Autodesk Inventor part; units mm, degrees
(part 4 of 8)
  line L1567 (12.2801, 87.4726) -> (12.299, 87.794) construction
  line L1568 (12.299, 87.794) -> (12.3274, 88.6686) construction
  line L1569 (12.3274, 88.6686) -> (12.3369, 89.0704) construction
  spline S407 degree 2 poles (9.1271, 85.2036) (9.6944, 85.2036) (10.3184, 86.0403) (10.3184, 86.8817) knots 0 0 0 1 2 2 2
  line L1570 (9.1271, 85.2036) -> (9.6944, 85.2036) construction
  line L1571 (9.6944, 85.2036) -> (10.3184, 86.0403) construction
  line L1572 (10.3184, 86.0403) -> (10.3184, 86.8817) construction
  spline S408 degree 2 poles (10.3184, 86.8817) (10.3184, 87.7326) (9.6991, 88.5599) (9.1271, 88.5599) knots 0 0 0 1 2 2 2
  line L1573 (10.3184, 86.8817) -> (10.3184, 87.7326) construction
  line L1574 (10.3184, 87.7326) -> (9.6991, 88.5599) construction
  line L1575 (9.6991, 88.5599) -> (9.1271, 88.5599) construction
  spline S409 degree 2 poles (9.1271, 88.5599) (8.5551, 88.5599) (7.9311, 87.7326) (7.9311, 86.8817) knots 0 0 0 1 2 2 2
  line L1576 (9.1271, 88.5599) -> (8.5551, 88.5599) construction
  line L1577 (8.5551, 88.5599) -> (7.9311, 87.7326) construction
  line L1578 (7.9311, 87.7326) -> (7.9311, 86.8817) construction
  spline S410 degree 2 poles (7.9311, 86.8817) (7.9311, 86.0544) (8.5551, 85.2036) (9.1271, 85.2036) knots 0 0 0 1 2 2 2
  line L1579 (7.9311, 86.8817) -> (7.9311, 86.0544) construction
  line L1580 (7.9311, 86.0544) -> (8.5551, 85.2036) construction
  line L1581 (8.5551, 85.2036) -> (9.1271, 85.2036) construction
  spline S411 degree 2 poles (9.1271, 84.5701) (8.2148, 84.5701) (7.1701, 85.8134) (7.1701, 86.8817) knots 0 0 0 1 2 2 2
  line L1582 (9.1271, 84.5701) -> (8.2148, 84.5701) construction
  line L1583 (8.2148, 84.5701) -> (7.1701, 85.8134) construction
  line L1584 (7.1701, 85.8134) -> (7.1701, 86.8817) construction
  spline S412 degree 2 poles (7.1701, 86.8817) (7.1701, 87.9784) (8.2478, 89.1933) (9.1271, 89.1933) knots 0 0 0 1 2 2 2
  line L1585 (7.1701, 86.8817) -> (7.1701, 87.9784) construction
  line L1586 (7.1701, 87.9784) -> (8.2478, 89.1933) construction
  line L1587 (8.2478, 89.1933) -> (9.1271, 89.1933) construction
  spline S413 degree 2 poles (9.1271, 89.1933) (10.0158, 89.1933) (11.0794, 87.9831) (11.0794, 86.8817) knots 0 0 0 1 2 2 2
  line L1588 (9.1271, 89.1933) -> (10.0158, 89.1933) construction
  line L1589 (10.0158, 89.1933) -> (11.0794, 87.9831) construction
  line L1590 (11.0794, 87.9831) -> (11.0794, 86.8817) construction
  spline S414 degree 2 poles (11.0794, 86.8817) (11.0794, 85.7755) (10.0158, 84.5701) (9.1271, 84.5701) knots 0 0 0 1 2 2 2
  line L1591 (11.0794, 86.8817) -> (11.0794, 85.7755) construction
  line L1592 (11.0794, 85.7755) -> (10.0158, 84.5701) construction
  line L1593 (10.0158, 84.5701) -> (9.1271, 84.5701) construction
  spline S415 degree 2 poles (4.7497, 85.2697) (5.3217, 85.2697) (5.9552, 86.1112) (5.9552, 86.9148) knots 0 0 0 1 2 2 2
  line L1594 (4.7497, 85.2697) -> (5.3217, 85.2697) construction
  line L1595 (5.3217, 85.2697) -> (5.9552, 86.1112) construction
  line L1596 (5.9552, 86.1112) -> (5.9552, 86.9148) construction
  spline S416 degree 2 poles (5.9552, 86.9148) (5.9552, 87.6664) (5.4777, 88.4937) (4.9436, 88.4937) knots 0 0 0 1 2 2 2
  line L1597 (5.9552, 86.9148) -> (5.9552, 87.6664) construction
  line L1598 (5.9552, 87.6664) -> (5.4777, 88.4937) construction
  line L1599 (5.4777, 88.4937) -> (4.9436, 88.4937) construction
  spline S417 degree 2 poles (4.9436, 88.4937) (4.6316, 88.4937) (4.0454, 88.2148) (3.7854, 87.9973) knots 0 0 0 1 2 2 2
  line L1600 (4.9436, 88.4937) -> (4.6316, 88.4937) construction
  line L1601 (4.6316, 88.4937) -> (4.0454, 88.2148) construction
  line L1602 (4.0454, 88.2148) -> (3.7854, 87.9973) construction
  line L1603 (3.7854, 87.9973) -> (3.7854, 85.5108)
  spline S418 degree 2 poles (3.7854, 85.5108) (4.0738, 85.3737) (4.485, 85.2697) (4.7497, 85.2697) knots 0 0 0 1 2 2 2
  line L1604 (3.7854, 85.5108) -> (4.0738, 85.3737) construction
  line L1605 (4.0738, 85.3737) -> (4.485, 85.2697) construction
  line L1606 (4.485, 85.2697) -> (4.7497, 85.2697) construction
  spline S419 degree 2 poles (4.8726, 84.6079) (4.5465, 84.6079) (4.0454, 84.7592) (3.7854, 84.9152) knots 0 0 0 1 2 2 2
  line L1607 (4.8726, 84.6079) -> (4.5465, 84.6079) construction
  line L1608 (4.5465, 84.6079) -> (4.0454, 84.7592) construction
  line L1609 (4.0454, 84.7592) -> (3.7854, 84.9152) construction
  spline S420 degree 2 poles (3.7854, 88.6119) (4.0596, 88.8624) (4.7308, 89.1933) (5.1232, 89.1933) knots 0 0 0 1 2 2 2
  line L1610 (3.7854, 88.6119) -> (4.0596, 88.8624) construction
  line L1611 (4.0596, 88.8624) -> (4.7308, 89.1933) construction
  line L1612 (4.7308, 89.1933) -> (5.1232, 89.1933) construction
  spline S421 degree 2 poles (5.1232, 89.1933) (5.8748, 89.1933) (6.7162, 88.002) (6.7162, 86.9999) knots 0 0 0 1 2 2 2
  line L1613 (5.1232, 89.1933) -> (5.8748, 89.1933) construction
  line L1614 (5.8748, 89.1933) -> (6.7162, 88.002) construction
  line L1615 (6.7162, 88.002) -> (6.7162, 86.9999) construction
  spline S422 degree 2 poles (6.7162, 86.9999) (6.7162, 85.9032) (5.6715, 84.6079) (4.8726, 84.6079) knots 0 0 0 1 2 2 2
  line L1616 (6.7162, 86.9999) -> (6.7162, 85.9032) construction
  line L1617 (6.7162, 85.9032) -> (5.6715, 84.6079) construction
  line L1618 (5.6715, 84.6079) -> (4.8726, 84.6079) construction
  spline S423 degree 2 poles (-7.9191, 85.2036) (-7.3518, 85.2036) (-6.7278, 86.0403) (-6.7278, 86.8817) knots 0 0 0 1 2 2 2
  line L1619 (-7.9191, 85.2036) -> (-7.3518, 85.2036) construction
  line L1620 (-7.3518, 85.2036) -> (-6.7278, 86.0403) construction
  line L1621 (-6.7278, 86.0403) -> (-6.7278, 86.8817) construction
  spline S424 degree 2 poles (-6.7278, 86.8817) (-6.7278, 87.7326) (-7.3471, 88.5599) (-7.9191, 88.5599) knots 0 0 0 1 2 2 2
  line L1622 (-6.7278, 86.8817) -> (-6.7278, 87.7326) construction
  line L1623 (-6.7278, 87.7326) -> (-7.3471, 88.5599) construction
  line L1624 (-7.3471, 88.5599) -> (-7.9191, 88.5599) construction
  spline S425 degree 2 poles (-7.9191, 88.5599) (-8.4911, 88.5599) (-9.1151, 87.7326) (-9.1151, 86.8817) knots 0 0 0 1 2 2 2
  line L1625 (-7.9191, 88.5599) -> (-8.4911, 88.5599) construction
  line L1626 (-8.4911, 88.5599) -> (-9.1151, 87.7326) construction
  line L1627 (-9.1151, 87.7326) -> (-9.1151, 86.8817) construction
  spline S426 degree 2 poles (-9.1151, 86.8817) (-9.1151, 86.0544) (-8.4911, 85.2036) (-7.9191, 85.2036) knots 0 0 0 1 2 2 2
  line L1628 (-9.1151, 86.8817) -> (-9.1151, 86.0544) construction
  line L1629 (-9.1151, 86.0544) -> (-8.4911, 85.2036) construction
  line L1630 (-8.4911, 85.2036) -> (-7.9191, 85.2036) construction
  spline S427 degree 2 poles (-7.9191, 84.5701) (-8.8314, 84.5701) (-9.8761, 85.8134) (-9.8761, 86.8817) knots 0 0 0 1 2 2 2
  line L1631 (-7.9191, 84.5701) -> (-8.8314, 84.5701) construction
  line L1632 (-8.8314, 84.5701) -> (-9.8761, 85.8134) construction
  line L1633 (-9.8761, 85.8134) -> (-9.8761, 86.8817) construction
  spline S428 degree 2 poles (-9.8761, 86.8817) (-9.8761, 87.9784) (-8.7983, 89.1933) (-7.9191, 89.1933) knots 0 0 0 1 2 2 2
  line L1634 (-9.8761, 86.8817) -> (-9.8761, 87.9784) construction
  line L1635 (-9.8761, 87.9784) -> (-8.7983, 89.1933) construction
  line L1636 (-8.7983, 89.1933) -> (-7.9191, 89.1933) construction
  spline S429 degree 2 poles (-7.9191, 89.1933) (-7.0304, 89.1933) (-5.9668, 87.9831) (-5.9668, 86.8817) knots 0 0 0 1 2 2 2
  line L1637 (-7.9191, 89.1933) -> (-7.0304, 89.1933) construction
  line L1638 (-7.0304, 89.1933) -> (-5.9668, 87.9831) construction
  line L1639 (-5.9668, 87.9831) -> (-5.9668, 86.8817) construction
  spline S430 degree 2 poles (-5.9668, 86.8817) (-5.9668, 85.7755) (-7.0304, 84.5701) (-7.9191, 84.5701) knots 0 0 0 1 2 2 2
  line L1640 (-5.9668, 86.8817) -> (-5.9668, 85.7755) construction
  line L1641 (-5.9668, 85.7755) -> (-7.0304, 84.5701) construction
  line L1642 (-7.0304, 84.5701) -> (-7.9191, 84.5701) construction
  spline S431 degree 2 poles (-1.6305, 79.8157) (-1.4362, 79.8157) (-1.3218, 79.944) knots 0 0 0 1 1 1
  line L1643 (-1.6305, 79.8157) -> (-1.4362, 79.8157) construction
  line L1644 (-1.4362, 79.8157) -> (-1.3218, 79.944) construction
  spline S432 degree 2 poles (-1.3218, 79.944) (-1.2177, 80.062) (-1.2177, 80.232) knots 0 0 0 1 1 1
  line L1645 (-1.3218, 79.944) -> (-1.2177, 80.062) construction
  line L1646 (-1.2177, 80.062) -> (-1.2177, 80.232) construction
  spline S433 degree 2 poles (-1.2177, 80.232) (-1.2177, 80.402) (-1.3218, 80.5165) knots 0 0 0 1 1 1
  line L1647 (-1.2177, 80.232) -> (-1.2177, 80.402) construction
  line L1648 (-1.2177, 80.402) -> (-1.3218, 80.5165) construction
  spline S434 degree 2 poles (-1.3218, 80.5165) (-1.4362, 80.6448) (-1.6305, 80.6448) knots 0 0 0 1 1 1
  line L1649 (-1.3218, 80.5165) -> (-1.4362, 80.6448) construction
  line L1650 (-1.4362, 80.6448) -> (-1.6305, 80.6448) construction
  spline S435 degree 2 poles (-1.6305, 81.0612) (-1.2385, 81.0612) (-1.0095, 80.801) knots 0 0 0 1 1 1
  line L1651 (-1.6305, 81.0612) -> (-1.2385, 81.0612) construction
  line L1652 (-1.2385, 81.0612) -> (-1.0095, 80.801) construction
  spline S436 degree 2 poles (-1.0095, 80.801) (-0.8014, 80.5685) (-0.8014, 80.232) knots 0 0 0 1 1 1
  line L1653 (-1.0095, 80.801) -> (-0.8014, 80.5685) construction
  line L1654 (-0.8014, 80.5685) -> (-0.8014, 80.232) construction
  spline S437 degree 2 poles (-0.8014, 80.232) (-0.8014, 79.8955) (-1.0095, 79.6561) knots 0 0 0 1 1 1
  line L1655 (-0.8014, 80.232) -> (-0.8014, 79.8955) construction
  line L1656 (-0.8014, 79.8955) -> (-1.0095, 79.6561) construction
  spline S438 degree 2 poles (-1.0095, 79.6561) (-1.2385, 79.3994) (-1.6305, 79.3994) knots 0 0 0 1 1 1
  line L1657 (-1.0095, 79.6561) -> (-1.2385, 79.3994) construction
  line L1658 (-1.2385, 79.3994) -> (-1.6305, 79.3994) construction
  line L1659 (-1.6305, 79.3994) -> (-2.255, 79.3994)
  spline S439 degree 2 poles (-2.255, 79.3994) (-2.4632, 79.3994) (-2.4632, 79.6075) knots 0 0 0 1 1 1
  line L1660 (-2.255, 79.3994) -> (-2.4632, 79.3994) construction
  line L1661 (-2.4632, 79.3994) -> (-2.4632, 79.6075) construction
  line L1662 (-2.4632, 79.6075) -> (-2.4632, 82.0985)
  spline S440 degree 2 poles (-2.4632, 82.0985) (-2.4632, 82.3067) (-2.255, 82.3067) knots 0 0 0 1 1 1
  line L1663 (-2.4632, 82.0985) -> (-2.4632, 82.3067) construction
  line L1664 (-2.4632, 82.3067) -> (-2.255, 82.3067) construction
  spline S441 degree 2 poles (-2.255, 82.3067) (-2.0468, 82.3067) (-2.0468, 82.0985) knots 0 0 0 1 1 1
  line L1665 (-2.255, 82.3067) -> (-2.0468, 82.3067) construction
  line L1666 (-2.0468, 82.3067) -> (-2.0468, 82.0985) construction
  spline S442 degree 2 poles (-12.0177, 79.6075) (-12.0177, 79.3994) (-12.2259, 79.3994) knots 0 0 0 1 1 1
  line L1667 (-12.0177, 79.6075) -> (-12.0177, 79.3994) construction
  line L1668 (-12.0177, 79.3994) -> (-12.2259, 79.3994) construction
  spline S443 degree 2 poles (-12.2259, 79.3994) (-12.434, 79.3994) (-12.434, 79.6075) knots 0 0 0 1 1 1
  line L1669 (-12.2259, 79.3994) -> (-12.434, 79.3994) construction
  line L1670 (-12.434, 79.3994) -> (-12.434, 79.6075) construction
  line L1671 (-12.434, 79.6075) -> (-12.434, 82.0985)
  spline S444 degree 2 poles (-12.434, 82.0985) (-12.434, 82.3067) (-12.2259, 82.3067) knots 0 0 0 1 1 1
  line L1672 (-12.434, 82.0985) -> (-12.434, 82.3067) construction
  line L1673 (-12.434, 82.3067) -> (-12.2259, 82.3067) construction
  line L1674 (-12.2259, 82.3067) -> (-10.3559, 82.3067)
  spline S445 degree 2 poles (-10.3559, 82.3067) (-10.0124, 82.3067) (-9.5267, 81.8209) (-9.5267, 81.4775) knots 0 0 0 1 2 2 2
  line L1675 (-10.3559, 82.3067) -> (-10.0124, 82.3067) construction
  line L1676 (-10.0124, 82.3067) -> (-9.5267, 81.8209) construction
  line L1677 (-9.5267, 81.8209) -> (-9.5267, 81.4775) construction
  line L1678 (-9.5267, 81.4775) -> (-9.5267, 79.6075)
  spline S446 degree 2 poles (-9.5267, 79.6075) (-9.5267, 79.3994) (-9.7349, 79.3994) knots 0 0 0 1 1 1
  line L1679 (-9.5267, 79.6075) -> (-9.5267, 79.3994) construction
  line L1680 (-9.5267, 79.3994) -> (-9.7349, 79.3994) construction
  spline S447 degree 2 poles (-9.7349, 79.3994) (-9.943, 79.3994) (-9.943, 79.6075) knots 0 0 0 1 1 1
  line L1681 (-9.7349, 79.3994) -> (-9.943, 79.3994) construction
  line L1682 (-9.943, 79.3994) -> (-9.943, 79.6075) construction
  line L1683 (-9.943, 79.6075) -> (-9.943, 81.474)
  spline S448 degree 2 poles (-9.943, 81.474) (-9.943, 81.644) (-10.1859, 81.8903) (-10.3559, 81.8903) knots 0 0 0 1 2 2 2
  line L1684 (-9.943, 81.474) -> (-9.943, 81.644) construction
  line L1685 (-9.943, 81.644) -> (-10.1859, 81.8903) construction
  line L1686 (-10.1859, 81.8903) -> (-10.3559, 81.8903) construction
  spline S449 degree 2 poles (-10.7722, 79.6075) (-10.7722, 79.3994) (-10.9804, 79.3994) knots 0 0 0 1 1 1
  line L1687 (-10.7722, 79.6075) -> (-10.7722, 79.3994) construction
  line L1688 (-10.7722, 79.3994) -> (-10.9804, 79.3994) construction
  spline S450 degree 2 poles (-10.9804, 79.3994) (-11.1885, 79.3994) (-11.1885, 79.6075) knots 0 0 0 1 1 1
  line L1689 (-10.9804, 79.3994) -> (-11.1885, 79.3994) construction
  line L1690 (-11.1885, 79.3994) -> (-11.1885, 79.6075) construction
  line L1691 (-15.9658, 79.3994) -> (-17.0031, 79.3994)
  spline S451 degree 2 poles (-17.0031, 79.3994) (-17.3431, 79.3994) (-17.8323, 79.8851) (-17.8323, 80.2285) knots 0 0 0 1 2 2 2
  line L1692 (-17.0031, 79.3994) -> (-17.3431, 79.3994) construction
  line L1693 (-17.3431, 79.3994) -> (-17.8323, 79.8851) construction
  line L1694 (-17.8323, 79.8851) -> (-17.8323, 80.2285) construction
  line L1695 (-17.8323, 80.2285) -> (-17.8323, 82.0985)
  spline S452 degree 2 poles (-17.8323, 82.0985) (-17.8323, 82.3067) (-17.6241, 82.3067) knots 0 0 0 1 1 1
  line L1696 (-17.8323, 82.0985) -> (-17.8323, 82.3067) construction
  line L1697 (-17.8323, 82.3067) -> (-17.6241, 82.3067) construction
  spline S453 degree 2 poles (-17.6241, 82.3067) (-17.416, 82.3067) (-17.416, 82.0985) knots 0 0 0 1 1 1
  line L1698 (-17.6241, 82.3067) -> (-17.416, 82.3067) construction
  line L1699 (-17.416, 82.3067) -> (-17.416, 82.0985) construction
  line L1700 (-17.416, 82.0985) -> (-17.416, 80.232)
  spline S454 degree 2 poles (-17.416, 80.232) (-17.416, 80.062) (-17.1731, 79.8157) (-17.0031, 79.8157) knots 0 0 0 1 2 2 2
  line L1701 (-17.416, 80.232) -> (-17.416, 80.062) construction
  line L1702 (-17.416, 80.062) -> (-17.1731, 79.8157) construction
  line L1703 (-17.1731, 79.8157) -> (-17.0031, 79.8157) construction
  spline S455 degree 2 poles (-16.174, 82.0985) (-16.174, 82.3067) (-15.9658, 82.3067) knots 0 0 0 1 1 1
  line L1704 (-16.174, 82.0985) -> (-16.174, 82.3067) construction
  line L1705 (-16.174, 82.3067) -> (-15.9658, 82.3067) construction
  spline S456 degree 2 poles (-15.9658, 82.3067) (-15.7576, 82.3067) (-15.7576, 82.0985) knots 0 0 0 1 1 1
  line L1706 (-15.9658, 82.3067) -> (-15.7576, 82.3067) construction
  line L1707 (-15.7576, 82.3067) -> (-15.7576, 82.0985) construction
  line L1708 (-15.7576, 82.0985) -> (-15.7576, 79.6075)
  spline S457 degree 2 poles (-15.7576, 79.6075) (-15.7576, 79.3994) (-15.9658, 79.3994) knots 0 0 0 1 1 1
  line L1709 (-15.7576, 79.6075) -> (-15.7576, 79.3994) construction
  line L1710 (-15.7576, 79.3994) -> (-15.9658, 79.3994) construction
  circle A68 centre (0.1742, -74.3888) radius 11.3681
  circle A69 centre (0.1742, -74.3888) radius 12.3682
  spline S458 degree 2 poles (-19.4906, 79.3994) (-19.8306, 79.3994) (-20.3233, 79.8851) (-20.3233, 80.2285) knots 0 0 0 1 2 2 2
  line L1711 (-19.4906, 79.3994) -> (-19.8306, 79.3994) construction
  line L1712 (-19.8306, 79.3994) -> (-20.3233, 79.8851) construction
  line L1713 (-20.3233, 79.8851) -> (-20.3233, 80.2285) construction
  line L1714 (-20.3233, 80.2285) -> (-20.3233, 81.4775)
  spline S459 degree 2 poles (-20.3233, 81.4775) (-20.3233, 81.8209) (-19.8306, 82.3067) (-19.4906, 82.3067) knots 0 0 0 1 2 2 2
  line L1715 (-20.3233, 81.4775) -> (-20.3233, 81.8209) construction
  line L1716 (-20.3233, 81.8209) -> (-19.8306, 82.3067) construction
  line L1717 (-19.8306, 82.3067) -> (-19.4906, 82.3067) construction
  line L1718 (-19.4906, 82.3067) -> (-18.8696, 82.3067)
  spline S460 degree 2 poles (-18.8696, 82.3067) (-18.6615, 82.3067) (-18.6615, 82.0985) knots 0 0 0 1 1 1
  line L1719 (-18.8696, 82.3067) -> (-18.6615, 82.3067) construction
  line L1720 (-18.6615, 82.3067) -> (-18.6615, 82.0985) construction
  spline S461 degree 2 poles (-18.6615, 82.0985) (-18.6615, 81.8903) (-18.8696, 81.8903) knots 0 0 0 1 1 1
  line L1721 (-18.6615, 82.0985) -> (-18.6615, 81.8903) construction
  line L1722 (-18.6615, 81.8903) -> (-18.8696, 81.8903) construction
  line L1723 (-18.8696, 81.8903) -> (-19.4906, 81.8903)
  spline S462 degree 2 poles (-19.4906, 81.8903) (-19.6606, 81.8903) (-19.907, 81.644) (-19.907, 81.474) knots 0 0 0 1 2 2 2
  line L1724 (-19.4906, 81.8903) -> (-19.6606, 81.8903) construction
  line L1725 (-19.6606, 81.8903) -> (-19.907, 81.644) construction
  line L1726 (-19.907, 81.644) -> (-19.907, 81.474) construction
  line L1727 (-19.907, 81.474) -> (-19.907, 80.232)
  spline S463 degree 2 poles (-19.907, 80.232) (-19.907, 80.062) (-19.6606, 79.8157) (-19.4906, 79.8157) knots 0 0 0 1 2 2 2
  line L1728 (-19.907, 80.232) -> (-19.907, 80.062) construction
  line L1729 (-19.907, 80.062) -> (-19.6606, 79.8157) construction
  line L1730 (-19.6606, 79.8157) -> (-19.4906, 79.8157) construction
  line L1731 (-19.4906, 79.8157) -> (-18.8696, 79.8157)
  spline S464 degree 2 poles (-18.8696, 79.8157) (-18.6615, 79.8157) (-18.6615, 79.6075) knots 0 0 0 1 1 1
  line L1732 (-18.8696, 79.8157) -> (-18.6615, 79.8157) construction
  line L1733 (-18.6615, 79.8157) -> (-18.6615, 79.6075) construction
  spline S465 degree 2 poles (-18.6615, 79.6075) (-18.6615, 79.3994) (-18.8696, 79.3994) knots 0 0 0 1 1 1
  line L1734 (-18.6615, 79.6075) -> (-18.6615, 79.3994) construction
  line L1735 (-18.6615, 79.3994) -> (-18.8696, 79.3994) construction
  line L1736 (-18.8696, 79.3994) -> (-19.4906, 79.3994)
  spline S466 degree 2 poles (-14.0924, 79.3994) (-14.4324, 79.3994) (-14.925, 79.8851) (-14.925, 80.2285) knots 0 0 0 1 2 2 2
  line L1737 (-14.0924, 79.3994) -> (-14.4324, 79.3994) construction
  line L1738 (-14.4324, 79.3994) -> (-14.925, 79.8851) construction
  line L1739 (-14.925, 79.8851) -> (-14.925, 80.2285) construction
  line L1740 (-14.925, 80.2285) -> (-14.925, 81.4775)
  spline S467 degree 2 poles (-14.925, 81.4775) (-14.925, 81.8209) (-14.4324, 82.3067) (-14.0924, 82.3067) knots 0 0 0 1 2 2 2
  line L1741 (-14.925, 81.4775) -> (-14.925, 81.8209) construction
  line L1742 (-14.925, 81.8209) -> (-14.4324, 82.3067) construction
  line L1743 (-14.4324, 82.3067) -> (-14.0924, 82.3067) construction
  line L1744 (-14.0924, 82.3067) -> (-13.4714, 82.3067)
  spline S468 degree 2 poles (-13.4714, 82.3067) (-13.2632, 82.3067) (-13.2632, 82.0985) knots 0 0 0 1 1 1
  line L1745 (-13.4714, 82.3067) -> (-13.2632, 82.3067) construction
  line L1746 (-13.2632, 82.3067) -> (-13.2632, 82.0985) construction
  spline S469 degree 2 poles (-13.2632, 82.0985) (-13.2632, 81.8903) (-13.4714, 81.8903) knots 0 0 0 1 1 1
  line L1747 (-13.2632, 82.0985) -> (-13.2632, 81.8903) construction
  line L1748 (-13.2632, 81.8903) -> (-13.4714, 81.8903) construction
  line L1749 (-13.4714, 81.8903) -> (-14.0924, 81.8903)
  spline S470 degree 2 poles (-14.0924, 81.8903) (-14.2624, 81.8903) (-14.5087, 81.644) (-14.5087, 81.474) knots 0 0 0 1 2 2 2
  line L1750 (-14.0924, 81.8903) -> (-14.2624, 81.8903) construction
  line L1751 (-14.2624, 81.8903) -> (-14.5087, 81.644) construction
  line L1752 (-14.5087, 81.644) -> (-14.5087, 81.474) construction
  line L1753 (-14.5087, 81.474) -> (-14.5087, 80.232)
  spline S471 degree 2 poles (-14.5087, 80.232) (-14.5087, 80.062) (-14.2624, 79.8157) (-14.0924, 79.8157) knots 0 0 0 1 2 2 2
  line L1754 (-14.5087, 80.232) -> (-14.5087, 80.062) construction
  line L1755 (-14.5087, 80.062) -> (-14.2624, 79.8157) construction
  line L1756 (-14.2624, 79.8157) -> (-14.0924, 79.8157) construction
  line L1757 (-14.0924, 79.8157) -> (-13.4714, 79.8157)
  spline S472 degree 2 poles (-13.4714, 79.8157) (-13.2632, 79.8157) (-13.2632, 79.6075) knots 0 0 0 1 1 1
  line L1758 (-13.4714, 79.8157) -> (-13.2632, 79.8157) construction
  line L1759 (-13.2632, 79.8157) -> (-13.2632, 79.6075) construction
  spline S473 degree 2 poles (-13.2632, 79.6075) (-13.2632, 79.3994) (-13.4714, 79.3994) knots 0 0 0 1 1 1
  line L1760 (-13.2632, 79.6075) -> (-13.2632, 79.3994) construction
  line L1761 (-13.2632, 79.3994) -> (-13.4714, 79.3994) construction
  line L1762 (-13.4714, 79.3994) -> (-14.0924, 79.3994)
  spline S474 degree 2 poles (-7.0357, 81.4775) (-7.0357, 81.6475) (-7.2786, 81.8903) (-7.4486, 81.8903) knots 0 0 0 1 2 2 2
  line L1763 (-7.0357, 81.4775) -> (-7.0357, 81.6475) construction
  line L1764 (-7.0357, 81.6475) -> (-7.2786, 81.8903) construction
  line L1765 (-7.2786, 81.8903) -> (-7.4486, 81.8903) construction
  line L1766 (-7.4486, 81.8903) -> (-7.8649, 81.8903)
  spline S475 degree 2 poles (-7.8649, 81.8903) (-8.0349, 81.8903) (-8.2778, 81.6475) (-8.2778, 81.4775) knots 0 0 0 1 2 2 2
  line L1767 (-7.8649, 81.8903) -> (-8.0349, 81.8903) construction
  line L1768 (-8.0349, 81.8903) -> (-8.2778, 81.6475) construction
  line L1769 (-8.2778, 81.6475) -> (-8.2778, 81.4775) construction
  spline S476 degree 2 poles (-8.2778, 80.232) (-8.2778, 80.062) (-8.0314, 79.8157) (-7.8614, 79.8157) knots 0 0 0 1 2 2 2
  line L1770 (-8.2778, 80.232) -> (-8.2778, 80.062) construction
  line L1771 (-8.2778, 80.062) -> (-8.0314, 79.8157) construction
  line L1772 (-8.0314, 79.8157) -> (-7.8614, 79.8157) construction
  line L1773 (-7.8614, 79.8157) -> (-6.8276, 79.8157)
  spline S477 degree 2 poles (-6.8276, 79.8157) (-6.6194, 79.8157) (-6.6194, 79.6075) knots 0 0 0 1 1 1
  line L1774 (-6.8276, 79.8157) -> (-6.6194, 79.8157) construction
  line L1775 (-6.6194, 79.8157) -> (-6.6194, 79.6075) construction
  spline S478 degree 2 poles (-6.6194, 79.6075) (-6.6194, 79.3994) (-6.8276, 79.3994) knots 0 0 0 1 1 1
  line L1776 (-6.6194, 79.6075) -> (-6.6194, 79.3994) construction
  line L1777 (-6.6194, 79.3994) -> (-6.8276, 79.3994) construction
  line L1778 (-6.8276, 79.3994) -> (-7.8649, 79.3994)
  spline S479 degree 2 poles (-7.8649, 79.3994) (-8.2084, 79.3994) (-8.6941, 79.8851) (-8.6941, 80.2285) knots 0 0 0 1 2 2 2
  line L1779 (-7.8649, 79.3994) -> (-8.2084, 79.3994) construction
  line L1780 (-8.2084, 79.3994) -> (-8.6941, 79.8851) construction
  line L1781 (-8.6941, 79.8851) -> (-8.6941, 80.2285) construction
  line L1782 (-8.6941, 80.2285) -> (-8.6941, 81.4775)
  spline S480 degree 2 poles (-8.6941, 81.4775) (-8.6941, 81.8209) (-8.2084, 82.3067) (-7.8649, 82.3067) knots 0 0 0 1 2 2 2
  line L1783 (-8.6941, 81.4775) -> (-8.6941, 81.8209) construction
  line L1784 (-8.6941, 81.8209) -> (-8.2084, 82.3067) construction
  line L1785 (-8.2084, 82.3067) -> (-7.8649, 82.3067) construction
  line L1786 (-7.8649, 82.3067) -> (-7.4486, 82.3067)
  spline S481 degree 2 poles (-7.4486, 82.3067) (-7.1051, 82.3067) (-6.6194, 81.8209) (-6.6194, 81.4775) knots 0 0 0 1 2 2 2
  line L1787 (-7.4486, 82.3067) -> (-7.1051, 82.3067) construction
  line L1788 (-7.1051, 82.3067) -> (-6.6194, 81.8209) construction
  line L1789 (-6.6194, 81.8209) -> (-6.6194, 81.4775) construction
  line L1790 (-6.6194, 81.4775) -> (-6.6194, 80.853)
  spline S482 degree 2 poles (-6.6194, 80.853) (-6.6194, 80.6448) (-6.8276, 80.6448) knots 0 0 0 1 1 1
  line L1791 (-6.6194, 80.853) -> (-6.6194, 80.6448) construction
  line L1792 (-6.6194, 80.6448) -> (-6.8276, 80.6448) construction
  spline S483 degree 2 poles (-3.504, 79.3994) (-3.7121, 79.3994) (-3.7121, 79.6075) knots 0 0 0 1 1 1
  line L1793 (-3.504, 79.3994) -> (-3.7121, 79.3994) construction
  line L1794 (-3.7121, 79.3994) -> (-3.7121, 79.6075) construction
  spline S484 degree 2 poles (-4.3713, 80.5269) (-4.4511, 80.4124) (-4.5413, 80.4124) knots 0 0 0 1 1 1
  line L1795 (-4.3713, 80.5269) -> (-4.4511, 80.4124) construction
  line L1796 (-4.4511, 80.4124) -> (-4.5413, 80.4124) construction
  spline S485 degree 2 poles (-4.5413, 80.4124) (-4.6315, 80.4124) (-4.7113, 80.5269) knots 0 0 0 1 1 1
  line L1797 (-4.5413, 80.4124) -> (-4.6315, 80.4124) construction
  line L1798 (-4.6315, 80.4124) -> (-4.7113, 80.5269) construction
  spline S486 degree 2 poles (-5.3705, 79.6075) (-5.3705, 79.3994) (-5.5786, 79.3994) knots 0 0 0 1 1 1
  line L1799 (-5.3705, 79.6075) -> (-5.3705, 79.3994) construction
  line L1800 (-5.3705, 79.3994) -> (-5.5786, 79.3994) construction
  spline S487 degree 2 poles (-5.5786, 79.3994) (-5.7868, 79.3994) (-5.7868, 79.6075) knots 0 0 0 1 1 1
  line L1801 (-5.5786, 79.3994) -> (-5.7868, 79.3994) construction
  line L1802 (-5.7868, 79.3994) -> (-5.7868, 79.6075) construction
  line L1803 (-5.7868, 79.6075) -> (-5.7868, 82.102)
  spline S488 degree 2 poles (-5.7868, 82.102) (-5.7868, 82.3413) (-5.6029, 82.3413) knots 0 0 0 1 1 1
  line L1804 (-5.7868, 82.102) -> (-5.7868, 82.3413) construction
  line L1805 (-5.7868, 82.3413) -> (-5.6029, 82.3413) construction
  spline S489 degree 2 poles (-5.6029, 82.3413) (-5.4954, 82.3413) (-5.4086, 82.2199) knots 0 0 0 1 1 1
  line L1806 (-5.6029, 82.3413) -> (-5.4954, 82.3413) construction
  line L1807 (-5.4954, 82.3413) -> (-5.4086, 82.2199) construction
  spline S490 degree 2 poles (-3.674, 82.2199) (-3.5872, 82.3413) (-3.4797, 82.3413) knots 0 0 0 1 1 1
  line L1808 (-3.674, 82.2199) -> (-3.5872, 82.3413) construction
  line L1809 (-3.5872, 82.3413) -> (-3.4797, 82.3413) construction
  spline S491 degree 2 poles (-3.4797, 82.3413) (-3.2958, 82.3413) (-3.2958, 82.102) knots 0 0 0 1 1 1
  line L1810 (-3.4797, 82.3413) -> (-3.2958, 82.3413) construction
  line L1811 (-3.2958, 82.3413) -> (-3.2958, 82.102) construction
  line L1812 (-3.2958, 82.102) -> (-3.2958, 79.6075)
  spline S492 degree 2 poles (-3.2958, 79.6075) (-3.2958, 79.3994) (-3.504, 79.3994) knots 0 0 0 1 1 1
  line L1813 (-3.2958, 79.6075) -> (-3.2958, 79.3994) construction
  line L1814 (-3.2958, 79.3994) -> (-3.504, 79.3994) construction
  spline S493 degree 2 poles (-0.1803, 79.3994) (-0.3885, 79.3994) (-0.3885, 79.6075) knots 0 0 0 1 1 1
  line L1815 (-0.1803, 79.3994) -> (-0.3885, 79.3994) construction
  line L1816 (-0.3885, 79.3994) -> (-0.3885, 79.6075) construction
  line L1817 (-0.3885, 79.6075) -> (-0.3885, 82.0985)
  spline S494 degree 2 poles (-0.3885, 82.0985) (-0.3885, 82.3067) (-0.1803, 82.3067) knots 0 0 0 1 1 1
  line L1818 (-0.3885, 82.0985) -> (-0.3885, 82.3067) construction
  line L1819 (-0.3885, 82.3067) -> (-0.1803, 82.3067) construction
  spline S495 degree 2 poles (-0.1803, 82.3067) (0.0278, 82.3067) (0.0278, 82.0985) knots 0 0 0 1 1 1
  line L1820 (-0.1803, 82.3067) -> (0.0278, 82.3067) construction
  line L1821 (0.0278, 82.3067) -> (0.0278, 82.0985) construction
  line L1822 (0.0278, 82.0985) -> (0.0278, 79.6075)
  spline S496 degree 2 poles (0.0278, 79.6075) (0.0278, 79.3994) (-0.1803, 79.3994) knots 0 0 0 1 1 1
  line L1823 (0.0278, 79.6075) -> (0.0278, 79.3994) construction
  line L1824 (0.0278, 79.3994) -> (-0.1803, 79.3994) construction
  spline S497 degree 2 poles (-12.8212, 87.1653) (-12.5375, 87.1701) (-12.1357, 87.4017) (-11.9939, 87.7326) knots 0 0 0 1 2 2 2
  line L1825 (-12.8212, 87.1653) -> (-12.5375, 87.1701) construction
  line L1826 (-12.5375, 87.1701) -> (-12.1357, 87.4017) construction
  line L1827 (-12.1357, 87.4017) -> (-11.9939, 87.7326) construction
  spline S498 degree 2 poles (-11.9939, 87.7326) (-11.9514, 87.8319) (-11.8474, 88.0919) (-11.8143, 88.1911) knots 0 0 0 1 2 2 2
  line L1828 (-11.9939, 87.7326) -> (-11.9514, 87.8319) construction
  line L1829 (-11.9514, 87.8319) -> (-11.8474, 88.0919) construction
  line L1830 (-11.8474, 88.0919) -> (-11.8143, 88.1911) construction
  spline S499 degree 2 poles (-11.8143, 88.1911) (-11.6441, 88.6733) (-11.0343, 89.0704) (-10.5427, 89.0704) knots 0 0 0 1 2 2 2
  line L1831 (-11.8143, 88.1911) -> (-11.6441, 88.6733) construction
  line L1832 (-11.6441, 88.6733) -> (-11.0343, 89.0704) construction
  line L1833 (-11.0343, 89.0704) -> (-10.5427, 89.0704) construction
  spline S500 degree 2 poles (-10.5143, 88.4369) (-10.8216, 88.4369) (-11.1288, 88.1817) (-11.2328, 87.8413) knots 0 0 0 1 2 2 2
  line L1834 (-10.5143, 88.4369) -> (-10.8216, 88.4369) construction
  line L1835 (-10.8216, 88.4369) -> (-11.1288, 88.1817) construction
  line L1836 (-11.1288, 88.1817) -> (-11.2328, 87.8413) construction
  spline S501 degree 2 poles (-11.2328, 87.8413) (-11.3416, 87.501) (-11.6394, 87.1228) (-11.819, 87.0188) knots 0 0 0 1 2 2 2
  line L1837 (-11.2328, 87.8413) -> (-11.3416, 87.501) construction
  line L1838 (-11.3416, 87.501) -> (-11.6394, 87.1228) construction
  line L1839 (-11.6394, 87.1228) -> (-11.819, 87.0188) construction
  spline S502 degree 2 poles (18.5342, 85.4399) (18.6902, 85.5439) (18.8367, 85.8181) (18.8367, 86.0355) knots 0 0 0 1 2 2 2
  line L1840 (18.5342, 85.4399) -> (18.6902, 85.5439) construction
  line L1841 (18.6902, 85.5439) -> (18.8367, 85.8181) construction
  line L1842 (18.8367, 85.8181) -> (18.8367, 86.0355) construction
  spline S503 degree 2 poles (18.8367, 86.0355) (18.8367, 86.2341) (18.6996, 86.5366) (18.5436, 86.6312) knots 0 0 0 1 2 2 2
  line L1843 (18.8367, 86.0355) -> (18.8367, 86.2341) construction
  line L1844 (18.8367, 86.2341) -> (18.6996, 86.5366) construction
  line L1845 (18.6996, 86.5366) -> (18.5436, 86.6312) construction
  spline S504 degree 2 poles (18.5436, 86.6312) (18.3782, 86.7304) (17.9622, 86.7683) (17.5746, 86.7683) knots 0 0 0 1 2 2 2
  line L1846 (18.5436, 86.6312) -> (18.3782, 86.7304) construction
  line L1847 (18.3782, 86.7304) -> (17.9622, 86.7683) construction
  line L1848 (17.9622, 86.7683) -> (17.5746, 86.7683) construction
  spline S505 degree 2 poles (17.5557, 85.2792) (17.948, 85.2792) (18.3782, 85.3454) (18.5342, 85.4399) knots 0 0 0 1 2 2 2
  line L1849 (17.5557, 85.2792) -> (17.948, 85.2792) construction
  line L1850 (17.948, 85.2792) -> (18.3782, 85.3454) construction
  line L1851 (18.3782, 85.3454) -> (18.5342, 85.4399) construction
  spline S506 degree 2 poles (19.1251, 85.0523) (18.8651, 84.8585) (18.2789, 84.693) (17.8204, 84.693) knots 0 0 0 1 2 2 2
  line L1852 (19.1251, 85.0523) -> (18.8651, 84.8585) construction
  line L1853 (18.8651, 84.8585) -> (18.2789, 84.693) construction
  line L1854 (18.2789, 84.693) -> (17.8204, 84.693) construction
  spline S507 degree 2 poles (17.8393, 87.3639) (18.3309, 87.3639) (18.8745, 87.2599) (19.144, 87.0613) knots 0 0 0 1 2 2 2
  line L1855 (17.8393, 87.3639) -> (18.3309, 87.3639) construction
  line L1856 (18.3309, 87.3639) -> (18.8745, 87.2599) construction
  line L1857 (18.8745, 87.2599) -> (19.144, 87.0613) construction
  spline S508 degree 2 poles (19.144, 87.0613) (19.3709, 86.8959) (19.5978, 86.3712) (19.5978, 86.0497) knots 0 0 0 1 2 2 2
  line L1858 (19.144, 87.0613) -> (19.3709, 86.8959) construction
  line L1859 (19.3709, 86.8959) -> (19.5978, 86.3712) construction
  line L1860 (19.5978, 86.3712) -> (19.5978, 86.0497) construction
  spline S509 degree 2 poles (19.5978, 86.0497) (19.5978, 85.733) (19.3425, 85.213) (19.1251, 85.0523) knots 0 0 0 1 2 2 2
  line L1861 (19.5978, 86.0497) -> (19.5978, 85.733) construction
  line L1862 (19.5978, 85.733) -> (19.3425, 85.213) construction
  line L1863 (19.3425, 85.213) -> (19.1251, 85.0523) construction
  spline S510 degree 2 poles (-16.8523, 41.3419) (-16.5089, 41.3419) (-16.0232, 41.8276) (-16.0232, 42.1711) knots 0 0 0 1 2 2 2
  line L1864 (-16.8523, 41.3419) -> (-16.5089, 41.3419) construction
  line L1865 (-16.5089, 41.3419) -> (-16.0232, 41.8276) construction
  line L1866 (-16.0232, 41.8276) -> (-16.0232, 42.1711) construction
  spline S511 degree 2 poles (-16.0232, 42.1711) (-16.0232, 42.5145) (-16.5089, 43.0002) (-16.8523, 43.0002) knots 0 0 0 1 2 2 2
  line L1867 (-16.0232, 42.1711) -> (-16.0232, 42.5145) construction
  line L1868 (-16.0232, 42.5145) -> (-16.5089, 43.0002) construction
  line L1869 (-16.5089, 43.0002) -> (-16.8523, 43.0002) construction
  spline S512 degree 2 poles (-17.6815, 39.4719) (-17.6815, 39.2638) (-17.8897, 39.2638) knots 0 0 0 1 1 1
  line L1870 (-17.6815, 39.4719) -> (-17.6815, 39.2638) construction
  line L1871 (-17.6815, 39.2638) -> (-17.8897, 39.2638) construction
  spline S513 degree 2 poles (-17.8897, 39.2638) (-18.0978, 39.2638) (-18.0978, 39.4719) knots 0 0 0 1 1 1
  line L1872 (-17.8897, 39.2638) -> (-18.0978, 39.2638) construction
  line L1873 (-18.0978, 39.2638) -> (-18.0978, 39.4719) construction
  line L1874 (-18.0978, 39.4719) -> (-18.0978, 43.2084)
  spline S514 degree 2 poles (-18.0978, 43.2084) (-18.0978, 43.2917) (-17.9729, 43.4166) (-17.8897, 43.4166) knots 0 0 0 1 2 2 2
  line L1875 (-18.0978, 43.2084) -> (-18.0978, 43.2917) construction
  line L1876 (-18.0978, 43.2917) -> (-17.9729, 43.4166) construction
  line L1877 (-17.9729, 43.4166) -> (-17.8897, 43.4166) construction
  line L1878 (-17.8897, 43.4166) -> (-16.8523, 43.4166)
  spline S515 degree 2 poles (-16.8523, 43.4166) (-16.3389, 43.4166) (-15.6069, 42.6845) (-15.6069, 42.1711) knots 0 0 0 1 2 2 2
  line L1879 (-16.8523, 43.4166) -> (-16.3389, 43.4166) construction
  line L1880 (-16.3389, 43.4166) -> (-15.6069, 42.6845) construction
  line L1881 (-15.6069, 42.6845) -> (-15.6069, 42.1711) construction
  spline S516 degree 2 poles (-15.6069, 42.1711) (-15.6069, 41.6576) (-16.3354, 40.9256) (-16.8523, 40.9256) knots 0 0 0 1 2 2 2
  line L1882 (-15.6069, 42.1711) -> (-15.6069, 41.6576) construction
  line L1883 (-15.6069, 41.6576) -> (-16.3354, 40.9256) construction
  line L1884 (-16.3354, 40.9256) -> (-16.8523, 40.9256) construction
  spline S517 degree 2 poles (-12.6996, 43.2188) (-12.6996, 43.427) (-12.4914, 43.427) knots 0 0 0 1 1 1
  line L1885 (-12.6996, 43.2188) -> (-12.6996, 43.427) construction
  line L1886 (-12.6996, 43.427) -> (-12.4914, 43.427) construction
  spline S518 degree 2 poles (-12.4914, 43.427) (-12.2832, 43.427) (-12.2832, 43.2188) knots 0 0 0 1 1 1
  line L1887 (-12.4914, 43.427) -> (-12.2832, 43.427) construction
  line L1888 (-12.2832, 43.427) -> (-12.2832, 43.2188) construction
  line L1889 (-12.2832, 43.2188) -> (-12.2832, 39.4789)
  spline S519 degree 2 poles (-12.2832, 39.4789) (-12.2832, 39.2672) (-12.4949, 39.2672) knots 0 0 0 1 1 1
  line L1890 (-12.2832, 39.4789) -> (-12.2832, 39.2672) construction
  line L1891 (-12.2832, 39.2672) -> (-12.4949, 39.2672) construction
  spline S520 degree 2 poles (-12.4949, 39.2672) (-12.6996, 39.2672) (-12.6996, 39.4719) knots 0 0 0 1 1 1
  line L1892 (-12.4949, 39.2672) -> (-12.6996, 39.2672) construction
  line L1893 (-12.6996, 39.2672) -> (-12.6996, 39.4719) construction
  spline S521 degree 2 poles (-14.3579, 39.4719) (-14.3579, 39.2638) (-14.5661, 39.2638) knots 0 0 0 1 1 1
  line L1894 (-14.3579, 39.4719) -> (-14.3579, 39.2638) construction
  line L1895 (-14.3579, 39.2638) -> (-14.5661, 39.2638) construction
  spline S522 degree 2 poles (-14.5661, 39.2638) (-14.7742, 39.2638) (-14.7742, 39.4719) knots 0 0 0 1 1 1
  line L1896 (-14.5661, 39.2638) -> (-14.7742, 39.2638) construction
  line L1897 (-14.7742, 39.2638) -> (-14.7742, 39.4719) construction
  line L1898 (-14.7742, 39.4719) -> (-14.7742, 43.2084)
  spline S523 degree 2 poles (-14.7742, 43.2084) (-14.7742, 43.4166) (-14.5661, 43.4166) knots 0 0 0 1 1 1
  line L1899 (-14.7742, 43.2084) -> (-14.7742, 43.4166) construction
  line L1900 (-14.7742, 43.4166) -> (-14.5661, 43.4166) construction
  spline S524 degree 2 poles (-14.5661, 43.4166) (-14.3579, 43.4166) (-14.3579, 43.2084) knots 0 0 0 1 1 1
  line L1901 (-14.5661, 43.4166) -> (-14.3579, 43.4166) construction
  line L1902 (-14.3579, 43.4166) -> (-14.3579, 43.2084) construction
  spline S525 degree 2 poles (-6.4382, 32.0286) (-6.8572, 32.0286) (-7.4497, 32.6212) (-7.4497, 33.0402) knots 0 0 0 1 2 2 2
  line L1903 (-6.4382, 32.0286) -> (-6.8572, 32.0286) construction
  line L1904 (-6.8572, 32.0286) -> (-7.4497, 32.6212) construction
  line L1905 (-7.4497, 32.6212) -> (-7.4497, 33.0402) construction
  line L1906 (-7.4497, 33.0402) -> (-7.4497, 34.8136)
  spline S526 degree 2 poles (-7.4497, 34.8136) (-7.4497, 35.0676) (-7.1958, 35.0676) knots 0 0 0 1 1 1
  line L1907 (-7.4497, 34.8136) -> (-7.4497, 35.0676) construction
  line L1908 (-7.4497, 35.0676) -> (-7.1958, 35.0676) construction
  spline S527 degree 2 poles (-7.1958, 35.0676) (-6.9418, 35.0676) (-6.9418, 34.8136) knots 0 0 0 1 1 1
  line L1909 (-7.1958, 35.0676) -> (-6.9418, 35.0676) construction
  line L1910 (-6.9418, 35.0676) -> (-6.9418, 34.8136) construction
  line L1911 (-6.9418, 34.8136) -> (-6.9418, 33.0444)
  spline S528 degree 2 poles (-6.9418, 33.0444) (-6.9418, 32.837) (-6.6413, 32.5365) (-6.4339, 32.5365) knots 0 0 0 1 2 2 2
  line L1912 (-6.9418, 33.0444) -> (-6.9418, 32.837) construction
  line L1913 (-6.9418, 32.837) -> (-6.6413, 32.5365) construction
  line L1914 (-6.6413, 32.5365) -> (-6.4339, 32.5365) construction
  spline S529 degree 2 poles (-4.9187, 34.8136) (-4.9187, 35.0676) (-4.6647, 35.0676) knots 0 0 0 1 1 1
  line L1915 (-4.9187, 34.8136) -> (-4.9187, 35.0676) construction
  line L1916 (-4.9187, 35.0676) -> (-4.6647, 35.0676) construction
  spline S530 degree 2 poles (-4.6647, 35.0676) (-4.4107, 35.0676) (-4.4107, 34.8136) knots 0 0 0 1 1 1
  line L1917 (-4.6647, 35.0676) -> (-4.4107, 35.0676) construction
  line L1918 (-4.4107, 35.0676) -> (-4.4107, 34.8136) construction
  line L1919 (-4.4107, 34.8136) -> (-4.4107, 31.0128)
  spline S531 degree 2 poles (-4.4107, 31.0128) (-4.4107, 30.5938) (-5.0033, 30.0012) (-5.4223, 30.0012) knots 0 0 0 1 2 2 2
  line L1920 (-4.4107, 31.0128) -> (-4.4107, 30.5938) construction
  line L1921 (-4.4107, 30.5938) -> (-5.0033, 30.0012) construction
  line L1922 (-5.0033, 30.0012) -> (-5.4223, 30.0012) construction
  line L1923 (-5.4223, 30.0012) -> (-6.6879, 30.0012)
  spline S532 degree 2 poles (-6.6879, 30.0012) (-6.9418, 30.0012) (-6.9418, 30.2551) knots 0 0 0 1 1 1
  line L1924 (-6.6879, 30.0012) -> (-6.9418, 30.0012) construction
  line L1925 (-6.9418, 30.0012) -> (-6.9418, 30.2551) construction
  spline S533 degree 2 poles (-6.9418, 30.2551) (-6.9418, 30.5091) (-6.6879, 30.5091) knots 0 0 0 1 1 1
  line L1926 (-6.9418, 30.2551) -> (-6.9418, 30.5091) construction
  line L1927 (-6.9418, 30.5091) -> (-6.6879, 30.5091) construction
  line L1928 (-6.6879, 30.5091) -> (-5.4223, 30.5091)
  spline S534 degree 2 poles (-5.4223, 30.5091) (-5.2149, 30.5091) (-4.9187, 30.8096) (-4.9187, 31.017) knots 0 0 0 1 2 2 2
  line L1929 (-5.4223, 30.5091) -> (-5.2149, 30.5091) construction
  line L1930 (-5.2149, 30.5091) -> (-4.9187, 30.8096) construction
  line L1931 (-4.9187, 30.8096) -> (-4.9187, 31.017) construction
  spline S535 degree 2 poles (-12.1271, 20.2534) (-11.7836, 20.2534) (-11.2979, 20.7391) (-11.2979, 21.0825) knots 0 0 0 1 2 2 2
  line L1932 (-12.1271, 20.2534) -> (-11.7836, 20.2534) construction
  line L1933 (-11.7836, 20.2534) -> (-11.2979, 20.7391) construction
  line L1934 (-11.2979, 20.7391) -> (-11.2979, 21.0825) construction
  spline S536 degree 2 poles (-11.2979, 21.0825) (-11.2979, 21.426) (-11.7836, 21.9117) (-12.1271, 21.9117) knots 0 0 0 1 2 2 2
  line L1935 (-11.2979, 21.0825) -> (-11.2979, 21.426) construction
  line L1936 (-11.2979, 21.426) -> (-11.7836, 21.9117) construction
  line L1937 (-11.7836, 21.9117) -> (-12.1271, 21.9117) construction
  spline S537 degree 2 poles (-12.9562, 18.3834) (-12.9562, 18.1752) (-13.1644, 18.1752) knots 0 0 0 1 1 1
  line L1938 (-12.9562, 18.3834) -> (-12.9562, 18.1752) construction
  line L1939 (-12.9562, 18.1752) -> (-13.1644, 18.1752) construction
  spline S538 degree 2 poles (-13.1644, 18.1752) (-13.3726, 18.1752) (-13.3726, 18.3834) knots 0 0 0 1 1 1
  line L1940 (-13.1644, 18.1752) -> (-13.3726, 18.1752) construction
  line L1941 (-13.3726, 18.1752) -> (-13.3726, 18.3834) construction
  line L1942 (-13.3726, 18.3834) -> (-13.3726, 22.1199)
  spline S539 degree 2 poles (-13.3726, 22.1199) (-13.3726, 22.2031) (-13.2477, 22.328) (-13.1644, 22.328) knots 0 0 0 1 2 2 2
  line L1943 (-13.3726, 22.1199) -> (-13.3726, 22.2031) construction
  line L1944 (-13.3726, 22.2031) -> (-13.2477, 22.328) construction
  line L1945 (-13.2477, 22.328) -> (-13.1644, 22.328) construction
  line L1946 (-13.1644, 22.328) -> (-12.1271, 22.328)
  spline S540 degree 2 poles (-12.1271, 22.328) (-11.6136, 22.328) (-10.8816, 21.596) (-10.8816, 21.0825) knots 0 0 0 1 2 2 2
  line L1947 (-12.1271, 22.328) -> (-11.6136, 22.328) construction
  line L1948 (-11.6136, 22.328) -> (-10.8816, 21.596) construction
  line L1949 (-10.8816, 21.596) -> (-10.8816, 21.0825) construction
  spline S541 degree 2 poles (-10.8816, 21.0825) (-10.8816, 20.5691) (-11.6101, 19.837) (-12.1271, 19.837) knots 0 0 0 1 2 2 2
  line L1950 (-10.8816, 21.0825) -> (-10.8816, 20.5691) construction
  line L1951 (-10.8816, 20.5691) -> (-11.6101, 19.837) construction
  line L1952 (-11.6101, 19.837) -> (-12.1271, 19.837) construction
  spline S542 degree 2 poles (-7.5927, 21.8111) (-7.5927, 21.7278) (-7.7175, 21.596) (-7.8008, 21.596) knots 0 0 0 1 2 2 2
  line L1953 (-7.5927, 21.8111) -> (-7.5927, 21.7278) construction
  line L1954 (-7.5927, 21.7278) -> (-7.7175, 21.596) construction
  line L1955 (-7.7175, 21.596) -> (-7.8008, 21.596) construction
  spline S543 degree 2 poles (-7.8008, 21.596) (-7.8667, 21.596) (-7.9257, 21.6376) knots 0 0 0 1 1 1
  line L1956 (-7.8008, 21.596) -> (-7.8667, 21.596) construction
  line L1957 (-7.8667, 21.596) -> (-7.9257, 21.6376) construction
  spline S544 degree 2 poles (-7.9257, 21.6376) (-8.3212, 21.9221) (-8.8034, 21.9221) knots 0 0 0 1 1 1
  line L1958 (-7.9257, 21.6376) -> (-8.3212, 21.9221) construction
  line L1959 (-8.3212, 21.9221) -> (-8.8034, 21.9221) construction
  spline S545 degree 2 poles (-8.8034, 21.9221) (-9.1157, 21.9221) (-9.6187, 21.6619) (-9.6187, 21.4121) knots 0 0 0 1 2 2 2
  line L1960 (-8.8034, 21.9221) -> (-9.1157, 21.9221) construction
  line L1961 (-9.1157, 21.9221) -> (-9.6187, 21.6619) construction
  line L1962 (-9.6187, 21.6619) -> (-9.6187, 21.4121) construction
  spline S546 degree 2 poles (-9.6187, 21.4121) (-9.6187, 21.2629) (-9.5008, 21.1727) knots 0 0 0 1 1 1
  line L1963 (-9.6187, 21.4121) -> (-9.6187, 21.2629) construction
  line L1964 (-9.6187, 21.2629) -> (-9.5008, 21.1727) construction
  line L1965 (-9.5008, 21.1727) -> (-7.9604, 20.0348)
  spline S547 degree 2 poles (-7.9604, 20.0348) (-7.5441, 19.7295) (-7.5441, 19.1813) knots 0 0 0 1 1 1
  line L1966 (-7.9604, 20.0348) -> (-7.5441, 19.7295) construction
  line L1967 (-7.5441, 19.7295) -> (-7.5441, 19.1813) construction
  spline S548 degree 2 poles (-7.5441, 19.1813) (-7.5441, 18.6124) (-8.4184, 18.1544) (-8.8381, 18.1544) knots 0 0 0 1 2 2 2
  line L1968 (-7.5441, 19.1813) -> (-7.5441, 18.6124) construction
  line L1969 (-7.5441, 18.6124) -> (-8.4184, 18.1544) construction
  line L1970 (-8.4184, 18.1544) -> (-8.8381, 18.1544) construction
  spline S549 degree 2 poles (-8.8381, 18.1544) (-9.3655, 18.1544) (-9.9379, 18.5256) knots 0 0 0 1 1 1
  line L1971 (-8.8381, 18.1544) -> (-9.3655, 18.1544) construction
  line L1972 (-9.3655, 18.1544) -> (-9.9379, 18.5256) construction
  spline S550 degree 2 poles (-9.9379, 18.5256) (-10.0351, 18.5881) (-10.0351, 18.6922) knots 0 0 0 1 1 1
  line L1973 (-9.9379, 18.5256) -> (-10.0351, 18.5881) construction
  line L1974 (-10.0351, 18.5881) -> (-10.0351, 18.6922) construction
  spline S551 degree 2 poles (-10.0351, 18.6922) (-10.0351, 18.7789) (-9.9136, 18.9107) (-9.8269, 18.9107) knots 0 0 0 1 2 2 2
  line L1975 (-10.0351, 18.6922) -> (-10.0351, 18.7789) construction
  line L1976 (-10.0351, 18.7789) -> (-9.9136, 18.9107) construction
  line L1977 (-9.9136, 18.9107) -> (-9.8269, 18.9107) construction
  spline S552 degree 2 poles (-9.8269, 18.9107) (-9.7679, 18.9107) (-9.7159, 18.8726) knots 0 0 0 1 1 1
  line L1978 (-9.8269, 18.9107) -> (-9.7679, 18.9107) construction
  line L1979 (-9.7679, 18.9107) -> (-9.7159, 18.8726) construction
  spline S553 degree 2 poles (-9.7159, 18.8726) (-9.2441, 18.5707) (-8.8277, 18.5707) knots 0 0 0 1 1 1
  line L1980 (-9.7159, 18.8726) -> (-9.2441, 18.5707) construction
  line L1981 (-9.2441, 18.5707) -> (-8.8277, 18.5707) construction
  spline S554 degree 2 poles (-8.8277, 18.5707) (-8.5086, 18.5707) (-8.172, 18.7442) knots 0 0 0 1 1 1
  line L1982 (-8.8277, 18.5707) -> (-8.5086, 18.5707) construction
  line L1983 (-8.5086, 18.5707) -> (-8.172, 18.7442) construction
  spline S555 degree 2 poles (-8.172, 18.7442) (-7.9465, 18.8656) (-7.9465, 19.1744) knots 0 0 0 1 1 1
  line L1984 (-8.172, 18.7442) -> (-7.9465, 18.8656) construction
  line L1985 (-7.9465, 18.8656) -> (-7.9465, 19.1744) construction
  spline S556 degree 2 poles (-7.9465, 19.1744) (-7.9465, 19.5109) (-8.1928, 19.6913) knots 0 0 0 1 1 1
  line L1986 (-7.9465, 19.1744) -> (-7.9465, 19.5109) construction
  line L1987 (-7.9465, 19.5109) -> (-8.1928, 19.6913) construction
  line L1988 (-8.1928, 19.6913) -> (-9.7332, 20.8327)
  spline S557 degree 2 poles (-9.7332, 20.8327) (-10.0177, 21.0409) (-10.0177, 21.4191) knots 0 0 0 1 1 1
  line L1989 (-9.7332, 20.8327) -> (-10.0177, 21.0409) construction
  line L1990 (-10.0177, 21.0409) -> (-10.0177, 21.4191) construction
  spline S558 degree 2 poles (-10.0177, 21.4191) (-10.0177, 21.9152) (-9.5563, 22.158) knots 0 0 0 1 1 1
  line L1991 (-10.0177, 21.4191) -> (-10.0177, 21.9152) construction
  line L1992 (-10.0177, 21.9152) -> (-9.5563, 22.158) construction
  spline S559 degree 2 poles (-9.5563, 22.158) (-9.2232, 22.328) (-8.8034, 22.328) knots 0 0 0 1 1 1
  line L1993 (-9.5563, 22.158) -> (-9.2232, 22.328) construction
  line L1994 (-9.2232, 22.328) -> (-8.8034, 22.328) construction
  spline S560 degree 2 poles (-8.8034, 22.328) (-8.179, 22.328) (-7.6863, 21.9776) knots 0 0 0 1 1 1
  line L1995 (-8.8034, 22.328) -> (-8.179, 22.328) construction
  line L1996 (-8.179, 22.328) -> (-7.6863, 21.9776) construction
  spline S561 degree 2 poles (-7.6863, 21.9776) (-7.5927, 21.9117) (-7.5927, 21.8111) knots 0 0 0 1 1 1
  line L1997 (-7.6863, 21.9776) -> (-7.5927, 21.9117) construction
  line L1998 (-7.5927, 21.9117) -> (-7.5927, 21.8111) construction
  spline S562 degree 2 poles (-10.9295, 16.7708) (-10.9295, 16.6875) (-11.0544, 16.5557) (-11.1377, 16.5557) knots 0 0 0 1 2 2 2
  line L1999 (-10.9295, 16.7708) -> (-10.9295, 16.6875) construction
  line L2000 (-10.9295, 16.6875) -> (-11.0544, 16.5557) construction
  line L2001 (-11.0544, 16.5557) -> (-11.1377, 16.5557) construction
  spline S563 degree 2 poles (-11.1377, 16.5557) (-11.2036, 16.5557) (-11.2626, 16.5973) knots 0 0 0 1 1 1
  line L2002 (-11.1377, 16.5557) -> (-11.2036, 16.5557) construction
  line L2003 (-11.2036, 16.5557) -> (-11.2626, 16.5973) construction
  spline S564 degree 2 poles (-11.2626, 16.5973) (-11.6581, 16.8818) (-12.1403, 16.8818) knots 0 0 0 1 1 1
  line L2004 (-11.2626, 16.5973) -> (-11.6581, 16.8818) construction
  line L2005 (-11.6581, 16.8818) -> (-12.1403, 16.8818) construction
  spline S565 degree 2 poles (-12.1403, 16.8818) (-12.4526, 16.8818) (-12.9556, 16.6216) (-12.9556, 16.3718) knots 0 0 0 1 2 2 2
  line L2006 (-12.1403, 16.8818) -> (-12.4526, 16.8818) construction
  line L2007 (-12.4526, 16.8818) -> (-12.9556, 16.6216) construction
  line L2008 (-12.9556, 16.6216) -> (-12.9556, 16.3718) construction
  spline S566 degree 2 poles (-12.9556, 16.3718) (-12.9556, 16.2226) (-12.8377, 16.1324) knots 0 0 0 1 1 1
  line L2009 (-12.9556, 16.3718) -> (-12.9556, 16.2226) construction
  line L2010 (-12.9556, 16.2226) -> (-12.8377, 16.1324) construction
  line L2011 (-12.8377, 16.1324) -> (-11.2973, 14.9945)
  spline S567 degree 2 poles (-11.2973, 14.9945) (-10.881, 14.6892) (-10.881, 14.141) knots 0 0 0 1 1 1
  line L2012 (-11.2973, 14.9945) -> (-10.881, 14.6892) construction
  line L2013 (-10.881, 14.6892) -> (-10.881, 14.141) construction
  spline S568 degree 2 poles (-10.881, 14.141) (-10.881, 13.572) (-11.7552, 13.1141) (-12.175, 13.1141) knots 0 0 0 1 2 2 2
  line L2014 (-10.881, 14.141) -> (-10.881, 13.572) construction
  line L2015 (-10.881, 13.572) -> (-11.7552, 13.1141) construction
  line L2016 (-11.7552, 13.1141) -> (-12.175, 13.1141) construction
  spline S569 degree 2 poles (-12.175, 13.1141) (-12.7024, 13.1141) (-13.2748, 13.4853) knots 0 0 0 1 1 1
  line L2017 (-12.175, 13.1141) -> (-12.7024, 13.1141) construction
  line L2018 (-12.7024, 13.1141) -> (-13.2748, 13.4853) construction
  spline S570 degree 2 poles (-13.2748, 13.4853) (-13.372, 13.5477) (-13.372, 13.6518) knots 0 0 0 1 1 1
  line L2019 (-13.2748, 13.4853) -> (-13.372, 13.5477) construction
  line L2020 (-13.372, 13.5477) -> (-13.372, 13.6518) construction
  spline S571 degree 2 poles (-13.372, 13.6518) (-13.372, 13.7386) (-13.2505, 13.8704) (-13.1638, 13.8704) knots 0 0 0 1 2 2 2
  line L2021 (-13.372, 13.6518) -> (-13.372, 13.7386) construction
  line L2022 (-13.372, 13.7386) -> (-13.2505, 13.8704) construction
  line L2023 (-13.2505, 13.8704) -> (-13.1638, 13.8704) construction
  spline S572 degree 2 poles (-13.1638, 13.8704) (-13.1048, 13.8704) (-13.0528, 13.8322) knots 0 0 0 1 1 1
  line L2024 (-13.1638, 13.8704) -> (-13.1048, 13.8704) construction
  line L2025 (-13.1048, 13.8704) -> (-13.0528, 13.8322) construction
  spline S573 degree 2 poles (-13.0528, 13.8322) (-12.581, 13.5304) (-12.1646, 13.5304) knots 0 0 0 1 1 1
  line L2026 (-13.0528, 13.8322) -> (-12.581, 13.5304) construction
  line L2027 (-12.581, 13.5304) -> (-12.1646, 13.5304) construction
  spline S574 degree 2 poles (-12.1646, 13.5304) (-11.8455, 13.5304) (-11.5089, 13.7039) knots 0 0 0 1 1 1
  line L2028 (-12.1646, 13.5304) -> (-11.8455, 13.5304) construction
  line L2029 (-11.8455, 13.5304) -> (-11.5089, 13.7039) construction